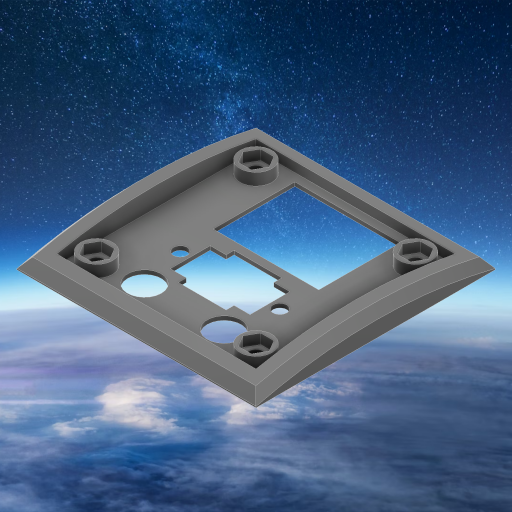
# Autodesk Inventor part: power_signal_socket
Saved by Autodesk Inventor 2023 (Build 270158000, 158)
## iProperties
Created: 2023-06-03
Part Number: power_signal_socket
Material: Acetal Resin, Black
Document SubType Name: Modeling
Designer: 310611102
Density: 1.425 g/cm^3
Appearance: Smooth - Black
Author: 310611102
Autodesk Inventor part; units mm, degrees
ref_plane "YZ Plane" through (0, 0, 0) normal (1, 0, 0) x (0, 1, 0)
ref_plane "XZ Plane" through (0, 0, 0) normal (0, 1, 0) x (-1, 0, 0)
sketch "Sketch1" plane through (0, 0, 0) normal (0, 1, 0) x (-1, 0, 0)
  line L0 (30, 30) -> (-30, 30)
  line L1 (-30, 30) -> (-30, -30)
  line L2 (-30, -30) -> (30, -30)
  line L3 (30, -30) -> (30, 30)
  line L4 (30, 30) -> (-30, -30) construction
  line L5 (-30, 30) -> (30, -30) construction
  point P0 (0, 0)
  dimension "d0" = 60
  dimension "d1" = 60
  constraints: 12 end point, 2 midpoint, 2 parallel, 1 horizontal, 1 perpendicular
  measures "d0" distance of L2.end L0.start
  measures "d1" distance of L1.end L2.end
extrude "Extrusion1" add sketch "Sketch1" along normal blind 6
sketch "Sketch2" plane through (30, 0, 30) normal (1, 0, 0) x (0, 0, -1)
  circle A0 centre (30, -119) radius 125
  line L0 (0, 6) -> (60, 6) projected
  line L1 (0, 0) -> (60, 0) projected
  point P0 (30, 0)
  point P1 (30, 0)
  dimension "d4" = 250
  constraints: 1 centre point, 1 midpoint, 1 tangent, 1 vertical alignment
  measures "d4" diameter of A0
extrude "Extrusion2" cut sketch "Sketch2" against normal through all keep common part
ref_plane "Work Plane1" through (30, 6, 0) normal (0, -1, 0) x (1, 0, 0)
sketch "Sketch3" plane through (30, 6, 0) normal (0, -1, 0) x (1, 0, 0)
  line L0 (-55, -25) -> (-5, -25)
  line L1 (-5, -25) -> (-5, 25)
  line L2 (-5, 25) -> (-55, 25)
  line L3 (-55, 25) -> (-55, -25)
  line L4 (-55, -25) -> (-5, 25) construction
  line L5 (-5, -25) -> (-55, 25) construction
  line L6 (0, -30) -> (-60, -30) projected
  line L7 (0, 30) -> (0, -30) projected
  point P0 (-30, 0)
  point P1 (-30, 0)
  dimension "d19" = 5
  dimension "d20" = 5
  constraints: 12 end point, 2 midpoint, 2 parallel, 1 coincident, 1 horizontal, 1 perpendicular
  measures "d19" distance between parallel lines of L6 L0
  measures "d20" distance between parallel lines of L7 L1
extrude "Extrusion3" cut sketch "Sketch3" along normal blind 5
sketch "Sketch4" plane through (30, 1, 0) normal (0, 1, 0) x (1, 0, 0)
  line L0 (-43.25, 23) -> (-16.75, 23)
  line L1 (-16.75, 23) -> (-16.75, 2.5)
  line L2 (-16.75, 2.5) -> (-43.25, 2.5)
  line L3 (-43.25, 2.5) -> (-43.25, 23)
  line L4 (-43.25, 23) -> (-16.75, 2.5) construction
  line L5 (-16.75, 23) -> (-43.25, 2.5) construction
  line L6 (-55, 25) -> (-5, 25) projected
  line L7 (-30, 12.75) -> (-30, 10.9588)
  line L8 (-40, -1.5) -> (-20, -1.5)
  line L9 (-20, -1.5) -> (-20, -11.5)
  line L10 (-20, -11.5) -> (-40, -11.5)
  line L11 (-40, -11.5) -> (-40, -1.5)
  line L12 (-40, -1.5) -> (-20, -11.5) construction
  line L13 (-20, -1.5) -> (-40, -11.5) construction
  circle A0 centre (-42.5, -6.5) radius 1.75
  circle A1 centre (-17.5, -6.5) radius 1.75
  circle A2 centre (-40, -18) radius 4.25
  circle A3 centre (-20, -18) radius 4.25
  line L14 (-24, -13.5) -> (-36, -13.5)
  line L15 (-36, -13.5) -> (-36, -11.5)
  line L16 (-36, -11.5) -> (-24, -11.5)
  line L17 (-24, -11.5) -> (-24, -13.5)
  line L18 (-24, -13.5) -> (-36, -11.5) construction
  line L19 (-36, -13.5) -> (-24, -11.5) construction
  line L20 (-24, 0.5) -> (-36, 0.5)
  line L21 (-36, 0.5) -> (-36, -1.5)
  line L22 (-36, -1.5) -> (-24, -1.5)
  line L23 (-24, -1.5) -> (-24, 0.5)
  line L24 (-24, 0.5) -> (-36, -1.5) construction
  line L25 (-36, 0.5) -> (-24, -1.5) construction
  line L26 (0, 30) -> (-60, 30) projected
  point P0 (-30, 0)
  point P1 (-30, -6.5)
  point P2 (-30, -12.5)
  point P3 (-30, -0.5)
  point P4 (-24, -11.5)
  point P5 (-24, -1.5)
  dimension "d11" = 20.5
  dimension "d12" = 26.5
  dimension "d13" = 2
  dimension "d26" = 10
  dimension "d27" = 20
  dimension "d28" = 4
  dimension "d29" = 3.5
  dimension "d30" = 3.5
  dimension "d31" = 25
  dimension "d38" = 8.5
  dimension "d42" = 20
  dimension "d43" = 12
  dimension "d44" = 2
  dimension "d45" = 12
  dimension "d46" = 2
  dimension "d64" = 48
  constraints: 50 end point, 14 point on line, 8 midpoint, 8 parallel, 4 centre point, 4 horizontal, 4 perpendicular, 4 vertical alignment, 2 horizontal alignment, 2 symmetric about line, 1 vertical, 1 other
  measures "d11" distance of L5.start L4.end
  measures "d12" distance of L4.start L5.start
  measures "d13" distance between parallel lines of L6 L0
  measures "d26" distance of L8.end L9.end
  measures "d27" distance of L8.start L8.end
  measures "d28" distance between parallel lines of L2 L8
  measures "d29" diameter of A0
  measures "d30" diameter of A1
  measures "d31" distance of A1.centre A0.centre
  measures "d38" diameter of A2
  measures "d42" distance of A3.centre A2.centre
  measures "d43" distance of L14.start L14.end
  measures "d44" distance of L16.end L14.start
  measures "d45" distance of L20.start L20.end
  measures "d46" distance of L20.end L21.end
  measures "d64" distance from line of L26 A2.centre
extrude "Extrusion4" cut sketch "Sketch4" against normal through all contours L0 L1 L2 L3
chamfer "Chamfer1" distance 2 angle 45 4 edges at (-30, 6, 0) (0, 2.3466, -30) (30, 6, 0) (0, 2.3466, 30)
extrude "Extrusion6" cut sketch "Sketch4" against normal blind 10 contours L8 L9 L10 L11 | L21 L20 L23 L8 | L10 L17 L14 L15
extrude "Extrusion7" cut sketch "Sketch4" against normal through all contours A0 | A1
sketch "Sketch8" plane through (30, 1, 0) normal (0, 1, 0) x (1, 0, 0)
  line L0 (-30, -21.9563) -> (-30, 0)
  line L1 (-30, 0) -> (-52.0851, 0)
  line L2 (-24, 0.5) -> (-36, 0.5) projected
  circle A0 centre (-10, -20) radius 4
  circle A1 centre (-50, -20) radius 4
  circle A2 centre (-10, 20) radius 4
  circle A3 centre (-50, 20) radius 4
  dimension "d56" = 8
  dimension "d57" = 40
  dimension "d58" = 40
  constraints: 4 centre point, 4 end point, 3 symmetric about line, 1 parallel, 1 vertical, 3 other
  measures "d56" diameter of A0
  measures "d57" diameter of A0.centre L0
  measures "d58" diameter of A0.centre L1
extrude "Extrusion11" add sketch "Sketch8" along normal blind 3
sketch "Sketch9" plane through (20, 4, 20) normal (0, 1, 0) x (1, 0, 0)
  circle A0 centre (0, 0) radius 4 projected
  line L0 (-3.2909, 0) -> (-1.6454, 2.85)
  line L1 (-1.6454, 2.85) -> (1.6454, 2.85)
  line L2 (1.6454, 2.85) -> (3.2909, 0)
  line L3 (3.2909, 0) -> (1.6454, -2.85)
  line L4 (1.6454, -2.85) -> (-1.6454, -2.85)
  line L5 (-1.6454, -2.85) -> (-3.2909, 0)
  line L6 (-20, 20) -> (-20, -14.7527)
  line L7 (-20, 20) -> (-56.1519, 20)
  line L8 (-36.7091, 0) -> (-38.3546, 2.85)
  line L9 (-38.3546, 2.85) -> (-41.6454, 2.85)
  line L10 (-41.6454, 2.85) -> (-43.2909, 0)
  line L11 (-43.2909, 0) -> (-41.6454, -2.85)
  line L12 (-41.6454, -2.85) -> (-38.3546, -2.85)
  line L13 (-38.3546, -2.85) -> (-36.7091, 0)
  line L14 (-3.2909, 40) -> (-1.6454, 37.15)
  line L15 (-1.6454, 37.15) -> (1.6454, 37.15)
  line L16 (1.6454, 37.15) -> (3.2909, 40)
  line L17 (3.2909, 40) -> (1.6454, 42.85)
  line L18 (1.6454, 42.85) -> (-1.6454, 42.85)
  line L19 (-1.6454, 42.85) -> (-3.2909, 40)
  line L20 (-43.2909, 40) -> (-41.6454, 42.85)
  line L21 (-41.6454, 42.85) -> (-38.3546, 42.85)
  line L22 (-38.3546, 42.85) -> (-36.7091, 40)
  line L23 (-36.7091, 40) -> (-38.3546, 37.15)
  line L24 (-38.3546, 37.15) -> (-41.6454, 37.15)
  line L25 (-41.6454, 37.15) -> (-43.2909, 40)
  dimension "d61" = 5.7
  constraints: 52 end point, 18 symmetric about line, 1 coincident, 1 horizontal, 1 horizontal alignment, 1 vertical, 13 other
  measures "d61" distance between parallel lines of L1 L4
extrude "Extrusion12" cut sketch "Sketch9" against normal blind 2.5 contours L0 L1 L2 L3 L4 L5 | L13 L12 L11 L10 L9 L8 | L19 L18 L17 L16 L15 L14 | L20 L21 L22 L23 L24 L25
extrude "Extrusion9" cut sketch "Sketch4" against normal through all contours A2 | A3
sketch "Sketch11" plane through (20, 1.5, 20) normal (0, 1, 0) x (1, 0, 0)
  circle A0 centre (0, 0) radius 1.75
  circle A1 centre (-40, 0) radius 1.75
  circle A2 centre (-40, 40) radius 1.75
  circle A3 centre (0, 40) radius 1.75
  point P0 (-20, 20)
  dimension "d72" = 3.5
  dimension "d73" = 3.5
  dimension "d74" = 3.5
  dimension "d75" = 3.5
  constraints: 4 centre point
  measures "d72" diameter of A0
  measures "d73" diameter of A1
  measures "d74" diameter of A2
  measures "d75" diameter of A3
extrude "Extrusion13" cut sketch "Sketch11" against normal through all
sketch "Sketch7" plane through (30, 1, 0) normal (0, 1, 0) x (1, 0, 0)
  circle A0 centre (-10, -6.5) radius 1.65
  circle A1 centre (-50, -6.5) radius 1.65
  line L0 (-30, -18.5284) -> (-30, 12.7052) construction
  circle A2 centre (-17.5, -6.5) radius 1.75 construction
  point P0 (-30, 0)
  dimension "d52" = 3.3
  dimension "d53" = 40
  constraints: 2 centre point, 2 end point, 1 horizontal alignment, 1 point on line, 1 vertical, 1 other
  measures "d52" diameter of A0
  measures "d53" distance of A1.centre A0.centre
equation "\"d30\" = d29"
equation "\"d45\" = d43"
equation "\"d46\" = d44"
equation "\"d73\" = d72"
equation "\"d74\" = d72"
equation "\"d75\" = d72"
body "Solid1"
